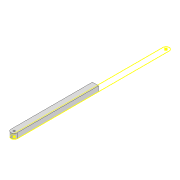
# Autodesk Inventor part: Part_12_p2
Saved by Autodesk Inventor 2022 (Build 260153000, 153)
## iProperties
Created: 2022-04-26
Part Number: Part_12_p2
Material: Generic
Document SubType Name: Modeling
Designer: dell
Density: 1 g/cm^3
Appearance: Default
Author: dell
Autodesk Inventor part; units mm, degrees
ref_plane "YZ Plane" through (0, 0, 0) normal (1, 0, 0) x (0, 1, 0)
ref_plane "XZ Plane" through (0, 0, 0) normal (0, 1, 0) x (-1, 0, 0)
ref_plane "XY Plane" through (0, 0, 0) normal (0, 0, 1) x (1, 0, 0)
sketch "Sketch1" plane through (0, 0, 0) normal (0, 1, 0) x (-1, 0, 0)
  line L0 (0, 0) -> (0, -244.795) construction
  line L1 (-5, 0) -> (-5, -244.795)
  line L2 (5, -244.795) -> (5, 0)
  arc A0 (5, 0) -> (-5, 0) centre (0, 0) ccw
  arc A1 (-5, -244.795) -> (5, -244.795) centre (0, -244.795) ccw
  circle A2 centre (0, 0) radius 1.5
  circle A3 centre (0, -244.795) radius 1.5
  point P0 (0, -122.3975)
  dimension "d0" = 244.795
  dimension "d1" = 10
  dimension "d2" = 3
  dimension "d3" = 3
  constraints: 8 end point, 4 centre point, 4 point on circle, 4 tangent, 2 coincident, 1 midpoint, 1 parallel, 1 vertical
  measures "d0" distance of L0.start L0.end
  measures "d1" diameter of A1
  measures "d2" diameter of A2
  measures "d3" diameter of A3
extrude "Extrusion1" add sketch "Sketch1" along normal blind 8
sketch "Sketch2" plane through (0, 8, 0) normal (0, 1, 0) x (1, 0, 0)
  arc A0 (5, 244.795) -> (-5, 244.795) centre (0, 244.795) ccw projected
  line L0 (-5, 244.795) -> (-5, 0) projected
  arc A1 (-5, 0) -> (5, 0) centre (0, 0) ccw projected
  line L1 (5, 0) -> (5, 244.795) projected
  circle A2 centre (0, 244.795) radius 1.5 projected
  circle A3 centre (0, 0) radius 1.5 projected
  circle A4 centre (0, 244.795) radius 5
  point P0 (-5, 244.795)
  dimension "d12" = 10
  constraints: 1 centre point, 1 coincident
  measures "d12" diameter of A4
extrude "Extrusion2" add sketch "Sketch2" along normal blind 12 contours A4 A0
sketch "Sketch3" plane through (0, 0, 0) normal (0, -1, 0) x (1, 0, 0)
  arc A0 (-5, -244.795) -> (5, -244.795) centre (0, -244.795) ccw projected
  line L0 (5, 0) -> (5, -244.795) projected
  arc A1 (5, 0) -> (-5, 0) centre (0, 0) ccw projected
  line L1 (-5, -244.795) -> (-5, 0) projected
  circle A2 centre (0, -244.795) radius 1.5 projected
  circle A3 centre (0, 0) radius 1.5 projected
sketch "Sketch4" plane through (0, 20, -244.795) normal (0, 1, 0) x (1, 0, 0)
  circle A0 centre (0, 0) radius 10
  point P0 (0, -244.795)
  dimension "d15" = 20
  constraints: 1 centre point
  measures "d15" diameter of A0
extrude "Extrusion3" add sketch "Sketch4" against normal blind 3
sketch "Sketch5" plane through (0, 0, 0) normal (0, -1, 0) x (1, 0, 0)
  line L0 (23.0807, 11.4027) -> (-31.8332, 11.4027)
  line L1 (-31.8332, 11.4027) -> (-31.8332, -131.2308)
  line L2 (-31.8332, -131.2308) -> (23.0807, -131.2308)
  line L3 (23.0807, -131.2308) -> (23.0807, 11.4027)
  line L4 (55.5298, 55.2625) -> (-102.4368, 55.2625)
  line L5 (-102.4368, 55.2625) -> (-102.4368, -369.4288)
  line L6 (-102.4368, -369.4288) -> (55.5298, -369.4288)
  line L7 (55.5298, -369.4288) -> (55.5298, 55.2625)
  point P0 (0, 0)
  constraints: 16 end point, 4 parallel, 2 horizontal, 2 perpendicular
extrude "Extrusion4" cut sketch "Sketch5" against normal blind 100
body "Solid1"
